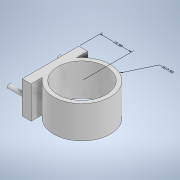
# Autodesk Inventor part: motor-hold
Saved by Autodesk Inventor 2022 (Build 260153000, 153)
## iProperties
Created: 2021-07-21
Part Number: motor-hold
Material: Generic
Document SubType Name: Modeling
Designer: WASHINGTON
Density: 1 g/cm^3
Appearance: Default
Author: WASHINGTON
Autodesk Inventor part; units mm, degrees
ref_plane "YZ Plane" through (0, 0, 0) normal (1, 0, 0) x (0, 1, 0)
ref_plane "XZ Plane" through (0, 0, 0) normal (0, 1, 0) x (-1, 0, 0)
ref_plane "XY Plane" through (0, 0, 0) normal (0, 0, 1) x (1, 0, 0)
sketch "Sketch1" plane through (0, 0, 0) normal (0, 1, 0) x (-1, 0, 0)
  circle A0 centre (0, 0) radius 15
  arc A1 (13.975, 10.5333) -> (13.975, -10.5333) centre (0, 0) ccw
  line L0 (13.975, 10.5333) -> (13.975, 17.5)
  line L1 (13.975, 17.5) -> (19.5, 17.5)
  line L2 (19.5, 17.5) -> (19.5, 0)
  line L3 (0, 0) -> (32.178, 0) construction
  line L4 (13.975, -10.5333) -> (13.975, -17.5)
  line L5 (13.975, -17.5) -> (19.5, -17.5)
  line L6 (19.5, -17.5) -> (19.5, 0)
  dimension "d0" = 30
  dimension "d2" = 19.5
  dimension "d3" = 17.5
  dimension "d4" = 5.525
  dimension "d5" = 13.975
  dimension "d6" = 35
  constraints: 14 end point, 3 symmetric about line, 2 centre point, 2 coincident, 2 point on circle, 2 vertical, 1 horizontal, 1 perpendicular
  measures "d0" diameter of A0
  measures "d2" distance of A0.centre L2.end
  measures "d3" distance of L1.end L2.end
  measures "d4" distance of L0.end L1.end
  measures "d5" distance from line of point (0, 0) L0
  measures "d6" diameter of A1
extrude "Extrusion1" add sketch "Sketch1" along normal mid plane 20
sketch "Sketch2" plane through (-19.5, -10, 17.5) normal (-1, 0, 0) x (0, 0, 1)
  circle A0 centre (-33, 10) radius 1.25
  circle A1 centre (-2, 10) radius 1.25
  line L0 (0, 0) -> (-35, 0) projected
  point P0 (-17.5, 10)
  dimension "d14" = 31
  dimension "d15" = 15.5
  dimension "d16" = 2.5
  dimension "d17" = 2.5
  dimension "d18" = 10
  dimension "d19" = 10
  constraints: 2 centre point
  measures "d14" distance of A1.centre A0.centre
  measures "d15" distance of A1.centre point (-17.5, 10)
  measures "d16" diameter of A1
  measures "d17" diameter of A0
  measures "d18" distance from line of L0 A1.centre
  measures "d19" distance from line of L0 A0.centre
extrude "Extrusion2" add sketch "Sketch2" along normal blind 10
body "Solid1"
